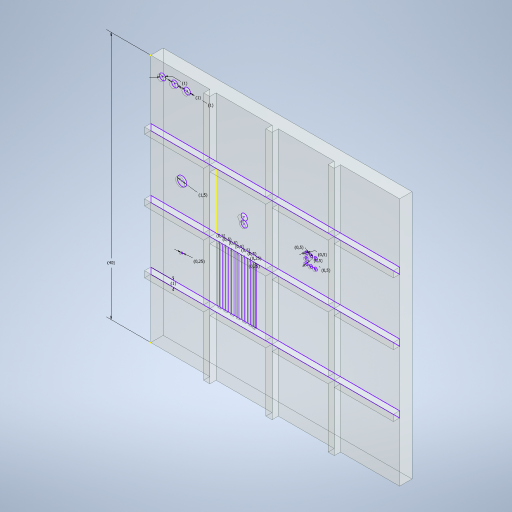
# Autodesk Inventor part: grating10
Saved by Autodesk Inventor 2023 (Build 270158000, 158)
## iProperties
Created: 2022-05-08
Part Number: grating10
Material: Glas
Document SubType Name: Sheet Metal
Designer: t1mst
Density: 2.18 g/cm^3
Sheet Metal Rule: Standard_mm
Appearance: Klar
Mass: 17.6144 g
Surface Area: 41.64 cm^2
Volume: 8.08 cm^3
Author: t1mst
Autodesk Inventor part; units mm, degrees
ref_plane "YZ Plane" through (0, 0, 0) normal (1, 0, 0) x (0, 1, 0)
ref_plane "XZ Plane" through (0, 0, 0) normal (0, 1, 0) x (-1, 0, 0)
ref_plane "XY Plane" through (0, 0, 0) normal (0, 0, 1) x (1, 0, 0)
sketch "Skizze1" plane through (0, 0, 0) normal (0, 0, 1) x (1, 0, 0)
  line L0 (0, 0) -> (0, 40)
  line L1 (0, 40) -> (40, 40)
  line L2 (40, 40) -> (40, 0)
  line L3 (40, 0) -> (0, 0)
  dimension "d0" = 40
  dimension "d1" = 40
  dimension "d2" = 40
  constraints: 8 end point, 2 vertical, 1 horizontal
  measures "d0" distance of L0.start L0.end
  measures "d1" distance of L0.end L1.end
  measures "d2" distance of L1.end L2.end
extrude "Extrusion1" add sketch "Skizze1" along normal blind 2
sketch "Skizze2" plane through (0, 0, 2) normal (0, 0, 1) x (1, 0, 0)
  line L0 (10.500065, 40) -> (10.500065, 0)
  line L1 (10.500065, 40) -> (9.500065, 40)
  line L2 (9.500065, 40) -> (9.500065, 0)
  line L3 (0, 0) -> (40, 0)
  line L4 (20.500065, 40) -> (20.500065, 0)
  line L5 (9.500065, 40) -> (10.500065, 40)
  line L6 (40, 40) -> (0, 40)
  line L7 (9.500065, 0) -> (10.500065, 0)
  dimension "d5" = 40
  dimension "d6" = 1
  constraints: 12 end point, 2 perpendicular, 2 point on line, 1 collinear, 1 horizontal, 1 vertical
  measures "d5" distance of L0.start L0.end
  measures "d6" distance of L0.start L1.end
extrude "Extrusion2" add sketch "Skizze2" along normal blind 1 contours L0 L3 L2 L1
sketch "Skizze3" plane through (0, 0, 2) normal (0, 0, 1) x (1, 0, 0)
  line L0 (20.500065, 40) -> (20.500065, 0)
  line L1 (20.500065, 40) -> (19.500065, 40)
  line L2 (40, 40) -> (10.500065, 40)
  line L3 (19.500065, 40) -> (19.500065, 0)
  line L4 (19.500065, 0) -> (20.500065, 0)
  line L5 (10.500065, 0) -> (40, 0)
  line L6 (19.500065, 40) -> (20.500065, 40)
  point P0 (0, 0)
  dimension "d11" = 40
  dimension "d12" = 1
  dimension "d13" = 40
  constraints: 10 end point, 2 collinear, 1 point on line
  measures "d11" distance of L0.start L0.end
  measures "d12" distance of L0.start L1.end
  measures "d13" distance of L1.end L3.end
extrude "Extrusion3" add sketch "Skizze3" along normal blind 1
sketch "Skizze4" plane through (0, 0, 2) normal (0, 0, 1) x (1, 0, 0)
  line L0 (29.5, 40) -> (30.5, 40)
  line L1 (30.5, 40) -> (30.5, 0)
  line L2 (0, 0) -> (40, 0) projected
  line L3 (29.5, 0) -> (29.5, 40)
  line L4 (29.5, 0) -> (30.5, 0)
  point P0 (40, 40)
  dimension "d17" = 1
  constraints: 8 end point, 2 perpendicular, 1 parallel, 1 point on line
  measures "d17" distance of L0.start L0.end
extrude "Extrusion4" add sketch "Skizze4" along normal blind 1
sketch "Skizze5" plane through (0, 0, 2) normal (0, 0, 1) x (1, 0, 0)
  line L0 (0, 30.5) -> (0, 29.5)
  line L1 (0, 30.5) -> (40, 30.5)
  line L2 (40, 29.5) -> (0, 29.5)
  line L3 (0, 20.5) -> (0, 19.5)
  line L4 (0, 19.5) -> (40, 19.5)
  line L5 (40, 20.5) -> (0, 20.5)
  line L6 (0, 9.5) -> (0, 10.5)
  line L7 (0, 10.5) -> (40, 10.5)
  line L8 (40, 9.5) -> (0, 9.5)
  line L9 (0, 30.5) -> (0, 29.5)
  line L10 (40, 30.5) -> (40, 29.5)
  line L11 (40, 20.5) -> (40, 19.5)
  line L12 (40, 10.5) -> (40, 9.5)
  line L13 (40, 30.5) -> (40, 29.5)
  point P0 (0, 0)
  point P1 (0, 40)
  dimension "d23" = 40
  dimension "d29" = 1
  constraints: 28 end point, 3 equal length, 2 vertical, 1 horizontal
  measures "d23" distance of point (0, 40) point (0, 0)
  measures "d29" distance of L6.start L6.end
extrude "Extrusion5" add sketch "Skizze5" along normal blind 1 contours L1 L10 L2 L0
sketch "Skizze6" plane through (0, 0, 2) normal (0, 0, 1) x (1, 0, 0)
  point P0 (0, 0)
extrude "Extrusion6" add sketch "Skizze5" along normal blind 1 contours L5 L11 L4 L3
extrude "Extrusion7" add sketch "Skizze5" along normal blind 1 contours L6 L7 L12 L8
sketch "Skizze7" plane through (0, 0, 2) normal (0, 0, 1) x (1, 0, 0)
  circle A0 centre (1.884735, 37.948882) radius 0.5
  circle A1 centre (3.849749, 37.948882) radius 0.5
  circle A2 centre (5.85748, 37.948882) radius 0.5
  line L0 (10.500065, 29.5) -> (19.500065, 29.5)
  line L1 (20.500065, 29.5) -> (29.5, 29.5)
  line L2 (19.500065, 19.5) -> (10.500065, 19.5)
  line L3 (20.500065, 19.5) -> (29.5, 19.5)
  line L4 (19.500065, 9.5) -> (10.500065, 9.5)
  line L5 (20.500065, 9.5) -> (29.5, 9.5)
  circle A3 centre (15.000065, 25) radius 0.5
  line L6 (10.500065, 20.5) -> (10.500065, 29.5)
  circle A4 centre (15.000065, 24) radius 0.5
  circle A5 centre (25.000032, 25) radius 0.25
  circle A6 centre (26.500032, 25) radius 0.25
  circle A7 centre (25.750032, 25) radius 0.25
  line L7 (25.000032, 23.5) -> (26.500032, 23.5)
  circle A8 centre (25.000032, 23.5) radius 0.25
  circle A9 centre (25.000032, 24.25) radius 0.25
  circle A10 centre (25.750032, 23.5) radius 0.25
  circle A11 centre (26.500032, 23.5) radius 0.25
  circle A12 centre (5.001314, 25) radius 0.75
  circle A13 centre (5.001314, 15) radius 0.125
  line L8 (11.012298, 19.5) -> (11.512298, 19.5)
  line L9 (11.512298, 19.5) -> (11.512298, 10.5)
  line L10 (10.500065, 10.5) -> (19.500065, 10.5)
  line L11 (11.512298, 10.5) -> (11.012298, 10.5)
  line L12 (11.012298, 19.5) -> (11.012298, 10.5)
  line L13 (12.012298, 19.495831) -> (12.512298, 19.495831)
  line L14 (12.512298, 19.495831) -> (12.512298, 10.495831)
  line L15 (12.512298, 10.495831) -> (12.012298, 10.495831)
  line L16 (12.012298, 19.495831) -> (12.012298, 10.495831)
  line L17 (12.998909, 19.505051) -> (12.998909, 10.505051)
  line L18 (13.498909, 19.505051) -> (13.498909, 10.505051)
  line L19 (13.498909, 10.505051) -> (12.998909, 10.505051)
  line L20 (12.998909, 19.505051) -> (13.498909, 19.505051)
  line L21 (14.012298, 19.500882) -> (14.012298, 10.500882)
  line L22 (14.512298, 19.500882) -> (14.512298, 10.500882)
  line L23 (14.512298, 10.500882) -> (14.012298, 10.500882)
  line L24 (14.012298, 19.500882) -> (14.512298, 19.500882)
  line L25 (15.012298, 19.496713) -> (15.012298, 10.496713)
  line L26 (15.512298, 19.496713) -> (15.512298, 10.496713)
  line L27 (15.512298, 10.496713) -> (15.012298, 10.496713)
  line L28 (15.012298, 19.496713) -> (15.512298, 19.496713)
  line L29 (16.012298, 19.505933) -> (16.012298, 10.505933)
  line L30 (16.512298, 19.505933) -> (16.512298, 10.505933)
  line L31 (16.512298, 10.505933) -> (16.012298, 10.505933)
  line L32 (16.012298, 19.505933) -> (16.512298, 19.505933)
  line L33 (10.500065, 19.5) -> (19.500065, 19.5)
  line L34 (16.762228, 19.5) -> (16.762228, 19.5)
  line L35 (16.762228, 19.5) -> (17.012228, 19.5)
  line L36 (17.012228, 19.5) -> (17.012228, 10.5)
  line L37 (17.012228, 10.5) -> (16.762228, 10.5)
  line L38 (19.500065, 10.5) -> (10.500065, 10.5)
  line L39 (16.762228, 19.5) -> (16.762228, 10.5)
  line L40 (16.762228, 19.5) -> (17.012228, 19.5)
  line L41 (16.762228, 10.5) -> (17.012228, 10.5)
  point P0 (0, 0)
  point P1 (12.012298, 10.5)
  point P2 (12.512298, 10.5)
  point P3 (13.498909, 19.5)
  point P4 (12.998909, 19.5)
  point P5 (15.012298, 10.5)
  point P6 (15.512298, 10.5)
  point P7 (16.512298, 19.5)
  point P8 (16.012298, 19.5)
  dimension "d36" = 1
  dimension "d37" = 1
  dimension "d38" = 1
  dimension "d46" = 0.5
  dimension "d48" = 0.5
  dimension "d49" = 0.5
  dimension "d50" = 0.5
  dimension "d51" = 1.5
  dimension "d52" = 0.25
  dimension "d53" = 0.5
  dimension "d54" = 0.5
  dimension "d55" = 0.5
  dimension "d56" = 0.5
  dimension "d57" = 0.5
  dimension "d58" = 0.5
  dimension "d99" = 0.25
  dimension "d100" = 0.25
  constraints: 64 end point, 14 centre point, 9 point on line, 8 perpendicular, 6 parallel, 2 coincident, 2 collinear, 1 equal radius, 1 midpoint
  measures "d36" diameter of A0
  measures "d37" diameter of A1
  measures "d38" diameter of A2
  measures "d46" diameter of A5
  measures "d48" diameter of A6
  measures "d49" diameter of A7
  measures "d50" diameter of A8
  measures "d51" diameter of A12
  measures "d52" diameter of A13
  measures "d53" distance of L8.start L8.end
  measures "d54" distance of L16.start L14.start
  measures "d55" distance of L20.start L20.end
  measures "d56" distance of L24.start L24.end
  measures "d57" distance of L28.start L28.end
  measures "d58" distance of L32.start L32.end
  measures "d99" distance of L32.end L34.start
  measures "d100" distance of L34.start L35.end
extrude "Extrusion8" add sketch "Skizze7" along normal blind 0.25 contours A12
extrude "Extrusion9" add sketch "Skizze7" along normal blind 0.25 contours L9 L10 L12 L2
extrude "Extrusion10" add sketch "Skizze7" along normal blind 0.25 contours L10 L16 L13 L14
extrude "Extrusion11" add sketch "Skizze7" along normal blind 0.25 contours L18 L19 L17 L2
sketch "Skizze7 outline for Extrusion12" plane through (0, 0, 2) normal (0, 0, 1) x (1, 0, 0)
  line L0 (14.012298, 10.500882) -> (14.512298, 10.500882)
  line L1 (14.012298, 19.500882) -> (14.012298, 10.500882)
  line L2 (14.512298, 19.500882) -> (14.012298, 19.500882)
  line L3 (14.512298, 10.500882) -> (14.512298, 19.500882)
extrude "Extrusion12" add sketch "Skizze7 outline for Extrusion12" along normal blind 0.25
extrude "Extrusion13" add sketch "Skizze7" along normal blind 0.25 contours L10 L25 L28 L26
extrude "Extrusion14" add sketch "Skizze7" along normal blind 0.25 contours L30 L31 L29 L2
extrude "Extrusion15" add sketch "Skizze7" along normal blind 0.25 contours A9
extrude "Extrusion16" add sketch "Skizze7" along normal blind 0.25 contours A8
extrude "Extrusion17" add sketch "Skizze7" along normal blind 0.25 contours A7
extrude "Extrusion18" add sketch "Skizze7" along normal blind 0.25 contours A5
extrude "Extrusion19" add sketch "Skizze7" along normal blind 0.25 contours A6
extrude "Extrusion20" add sketch "Skizze7" along normal blind 0.25 contours A11
extrude "Extrusion21" add sketch "Skizze7" along normal blind 0.25 contours A10 L7 | L7 A10
extrude "Extrusion22" add sketch "Skizze7" along normal blind 0.25 contours A13
extrude "Extrusion23" add sketch "Skizze7" along normal blind 0.5 contours A3
extrude "Extrusion24" add sketch "Skizze7" along normal blind 0.25 contours A4
extrude "Extrusion25" add sketch "Skizze7" along normal blind 0.35 contours A0
extrude "Extrusion26" add sketch "Skizze7" along normal blind 0.35 contours A1
extrude "Extrusion27" add sketch "Skizze7" along normal blind 0.35 contours A2
extrude "Extrusion28" add sketch "Skizze7" along normal blind 0.35 contours L36 L10 L39 L2
equation "\"Biegeradius\" = Stärke"
equation "\"BreiteBiegungsfreistellung\" = Stärke"
equation "\"TiefeBiegungsfreistellung\" = 0.5 * Stärke"
equation "\"GrößeEckenfreistellung\" = 4 * Stärke"
equation "\"MinimalRest\" = 2 * Stärke"
equation "\"Übergangsradius\" = Biegeradius"
equation "\"JacobiRadiusGröße\" = Biegeradius"
equation "\"Abstandsgröße\" = Stärke"
equation "\"Stärke\" = 0.5"
